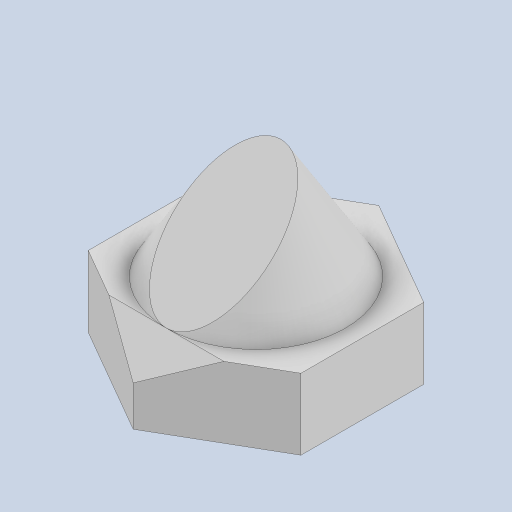
# Autodesk Inventor part: Санёк
Saved by Autodesk Inventor 2024 (Build 280153000, 153)
## iProperties
Created: 2023-12-09
Part Number: Санёк
Material: Типовые
Document SubType Name: Modeling
Designer: User
Density: 1 g/cm^3
Appearance: По умолчанию
Author: User
Autodesk Inventor part; units mm, degrees
ref_plane "YZ Plane" through (0, 0, 0) normal (1, 0, 0) x (0, 1, 0)
ref_plane "XZ Plane" through (0, 0, 0) normal (0, 1, 0) x (-1, 0, 0)
sketch "Эскиз1" plane through (0, 0, 0) normal (0, 1, 0) x (-1, 0, 0)
  line L0 (0, -34.6222) -> (-29.9837, -17.3111)
  line L1 (-29.9837, -17.3111) -> (-29.9837, 17.3111)
  line L2 (-29.9837, 17.3111) -> (0, 34.6222)
  line L3 (0, 34.6222) -> (29.9837, 17.3111)
  line L4 (29.9837, 17.3111) -> (29.9837, -17.3111)
  line L5 (29.9837, -17.3111) -> (0, -34.6222)
  point P0 (0, 0)
  point P1 (0, 0)
  constraints: 12 end point, 13 other
extrude "Выдавливание1" add sketch "Эскиз1" against normal blind 20
sketch "Эскиз2" plane through (0, 0, 0) normal (0, 1, 0) x (1, 0, 0)
  circle A0 centre (0, 0) radius 25.2598
  constraints: 1 centre point, 1 coincident
ref_plane "РабПлоскость2" through (0, 41.5, 0) normal (0, 1, 0) x (1, 0, 0)
sketch "Эскиз3" plane through (0, 41.5, 0) normal (0, 1, 0) x (1, 0, 0)
  point P0 (0, 0)
  point P1 (0, 0)
  constraints: 1 coincident
loft "Лофт1" add profiles "Эскиз2" section 1 point at (0, 41.5, 0)
sketch "Эскиз4" plane through (0, 0, 0) normal (1, 0, 0) x (0, 1, 0)
  line L0 (-20, 17.3111) -> (-20, -17.3111) projected
  line L1 (0, -25.2598) -> (41.5, 0) projected
  line L2 (29.9669, -7.0199) -> (0, 25.2598)
  line L3 (0, 25.2598) -> (41.5, 0) projected
  line L4 (0, 25.2598) -> (-8.6916, 34.6222)
  line L5 (0, 17.3111) -> (0, 34.6222) projected
  line L6 (-8.6916, 34.6222) -> (0, 34.6222)
  line L7 (0, 34.6222) -> (29.9669, 34.6222)
  line L8 (29.9669, 34.6222) -> (52.4176, 17.3111)
  line L9 (52.4176, 17.3111) -> (52.4176, -10.8837)
  arc A0 (29.9669, -7.0199) -> (52.4176, -10.8837) centre (52.4176, 56.2726) ccw
  point P0 (0, 0)
  constraints: 12 end point, 5 point on line, 2 perpendicular, 2 point on circle, 1 centre point
extrude "Выдавливание2" cut sketch "Эскиз4" along normal mid plane 535
